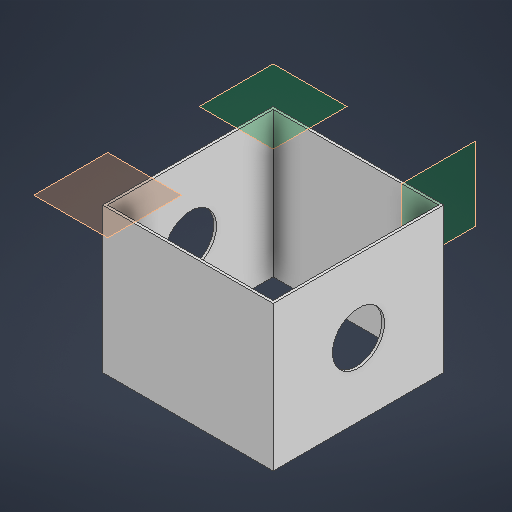
# Autodesk Inventor part: Container
Saved by Autodesk Inventor 2026 (Build 300175050, 175E)
## iProperties
Created: 2025-11-03
Part Number: Container
Material: Generic
Document SubType Name: Modeling
Designer: randy
Density: 1 g/cm^3
Appearance: Default
Author: randy
Autodesk Inventor part; units mm, degrees
ref_plane "YZ Plane" through (0, 0, 0) normal (1, 0, 0) x (0, 1, 0)
ref_plane "XY Plane" through (0, 0, 0) normal (0, 0, 1) x (1, 0, 0)
ref_plane "Work Plane1" through (0, -25.4, 0) normal (0, 1, 0) x (-1, 0, 0)
ref_plane "Work Plane2" through (-24.6309, -22.86, 24.6309) normal (0, 1, 0) x (1, 0, 0)
ref_plane "Work Plane3" through (24.6309, -25.4, -24.6309) normal (-1, 0, 0) x (0, 0, 1)
sketch "Sketch6" plane through (24.6309, -25.4, -24.6309) normal (-1, 0, 0) x (0, 0, 1)
  line L0 (0, 0) -> (0, -43.18)
  line L1 (49.2619, 0) -> (49.2619, -43.18)
  circle A0 centre (24.6309, -21.5887) radius 12.7 construction
  line L2 (11.9309, -21.5887) -> (3.0409, -21.5887) construction
  line L3 (24.6309, -8.8887) -> (24.6309, 0.0013) construction
  line L4 (49.2619, -21.5887) -> (60.6073, -21.5887) construction
  line L5 (24.6309, -34.2887) -> (24.6309, -43.1787) construction
  line L6 (-8.214, 0) -> (61.3562, 0)
  point P0 (24.6309, 25.4)
  point P1 (24.6309, 0)
  dimension "d30" = 25.4
  dimension "d39" = 11.3454
  dimension "d42" = 8.89
  dimension "d43" = 8.89
  dimension "d45" = 8.89
  dimension "d46" = 43.18
  dimension "d57" = 8.214
  constraints: 14 end point, 4 vertical, 3 point on circle, 2 horizontal, 2 horizontal alignment, 1 centre point, 1 perpendicular, 1 point on line, 1 vertical alignment
  measures "d30" diameter of A0
  measures "d39" distance from line of L1 L4.end
  measures "d42" distance of L2.start L2.end
  measures "d43" distance of L3.start L3.end
  measures "d45" distance of L5.start L5.end
  measures "d46" distance of L0.start L0.end
  measures "d57" distance of L0.start L6.start
ref_plane "Work Plane5" through (-25.4, -25.4, -25.4) normal (0, -1, 0) x (1, 0, 0)
sketch "Sketch7" plane through (-25.4, -25.4, -25.4) normal (0, -1, 0) x (1, 0, 0)
  line L0 (0.7691, 50.0309) -> (50.0309, 50.0309) projected
  line L1 (50.0309, 50.0309) -> (50.0309, 0.7691) projected
  line L2 (50.0309, 0.7691) -> (0.7691, 0.7691) projected
  line L3 (0.7691, 0.7691) -> (0.7691, 50.0309) projected
  line L4 (0, 50.8) -> (0, 0) projected
  line L5 (0, 0) -> (50.8, 0) projected
  line L6 (50.8, 0) -> (50.8, 50.8) projected
  line L7 (50.8, 50.8) -> (0, 50.8) projected
  point P0 (25.4, 25.4)
extrude "Extrusion3" add sketch "Sketch7" along normal blind 43.18
sketch "Sketch8" plane through (-25.4, -68.58, -25.4) normal (-1, 0, 0) x (0, 0, 1)
  line L0 (50.8, 43.18) -> (0, 43.18) projected
  line L1 (0, 43.18) -> (0, 0) projected
  line L2 (50.8, 0) -> (0, 0) projected
  line L3 (50.8, 43.18) -> (50.8, 0) projected
  circle A0 centre (25.4, 21.59) radius 7.747
  point P0 (25.4, 68.58)
  dimension "d54" = 15.494
  dimension "d55" = 21.59
  dimension "d56" = 25.4
  constraints: 1 centre point
  measures "d54" diameter of A0
  measures "d55" distance from line of L0 A0.centre
  measures "d56" distance from line of L1 A0.centre
extrude "Extrusion4" cut sketch "Sketch8" along normal through all both and the other way through all contours A0
equation "\"d43\" = d42"
equation "\"d45\" = d42"
body "Solid1"
